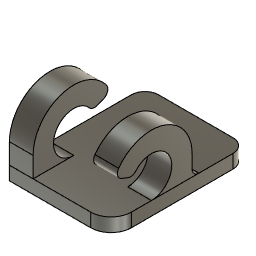
CableGuide v3 (Autodesk Fusion 360 design; units mm, degrees)
Autodesk Fusion 360 part; units mm, degrees
note: some values were not read from the file. Set by a fixed rule: which sketch regions a step uses.
sketch "Sketch1" plane through (0, 0, 0) normal (0, 0, 1) x (1, 0, 0)
  line L0 (-32.9657, 43.8587) -> (-17.9657, 43.8587)
  line L1 (-17.9657, 43.8587) -> (-17.9657, 23.8587)
  line L2 (-17.9657, 23.8587) -> (-32.9657, 23.8587)
  line L3 (-32.9657, 23.8587) -> (-32.9657, 43.8587)
  circle A0 centre (-25.4657, 38.8587) radius 2
  dimension "d1" = 15
  dimension "d2" = 20
  dimension "d3" = 4
  dimension "d4" = 7.5
  dimension "d5" = 5
  constraint horizontal L0
  constraint vertical L1
  constraint horizontal L2
  constraint vertical L3
  measures "d1" distance of L0.start L0.end
  measures "d2" distance of L0.start L2.end
  measures "d3" diameter of A0
  measures "d4" distance of L1 A0.centre
  measures "d5" distance of L0 A0.centre
extrude "Extrude1" add sketch "Sketch1" along normal blind 2 makes body 1
sketch "Sketch3" plane through (0, 0, 0) normal (1, 0, 0) x (0, 1, 0)
  circle A0 centre (27.5, 5) radius 3
  circle A1 centre (27.5, 5) radius 6
  line L0 (24.8198, 6.3478) -> (22.0216, 7.4469)
  line L1 (33.5, 5) -> (33.5, 2)
  line L2 (33.5, 2) -> (27.5, 2)
  constraint concentric A0 A1
  constraint coincident A0 L0.start
  constraint coincident A1 L0.end
  constraint coincident A1 L1.start
  constraint tangent A1 L1
  constraint vertical L1
  constraint coincident A0 L2.end
  constraint tangent A0 L2
  constraint perpendicular L1 L2
extrude "Extrude3" add sketch "Sketch3" along normal blind 3.5 separate body contours A0 A1 L0 L2 | A1 L1 L2 picked at (25.7298, 9.6652) makes body 2
move_body "Move6" bodies 2 to x (1, 0, 0) y (0, 1, 0) z (0, 0, 1) at (-22, 2, 0)
move_body "Move7" bodies 2 to x (1, 0, 0) y (0, 1, 0) z (0, 0, 1) at (0.5, 0, 0)
copy_body "CopyPasteBodies2" bodies 2 makes body 3
move_body "Move8" bodies 3 to x (-1, 0, 0) y (0, -1, 0) z (0, 0, 1) at (-52, 48.0432, 0)
move_body "Move9" bodies 3 to x (1, 0, 0) y (0, 1, 0) z (0, 0, 1) at (0, 11, 0)
move_body "Move10" bodies 3 to x (1, 0, 0) y (0, 1, 0) z (0, 0, 1) at (1, 0, 0)
move_body "Move11" bodies 3 to x (1, 0, 0) y (0, 1, 0) z (0, 0, 1) at (0.034, 0, 0)
move_body "Move12" bodies 2 to x (1, 0, 0) y (0, 1, 0) z (0, 0, 1) at (0.034, 0, 0)
move_body "Move13" bodies 2 3 to x (1, 0, 0) y (0, 1, 0) z (0, 0, 1) at (0, 0.316, 0)
combine "Combine2" operation add target body 3 tool bodies 2 1
fillet "Fillet6" radius 3 1 edges at (-17.9657, 23.8587, 1) on bodies 3
fillet "Fillet7" radius 2 2 edges at (-17.9657, 43.8587, 1) (-32.9657, 43.8587, 1) on bodies 3
fillet "Fillet8" radius 1 2 edges at (-19.716, 27.1358, 6.3478) (-19.716, 24.3376, 7.4469) on bodies 3
fillet "Fillet9" radius 1 2 edges at (-31.216, 32.5394, 6.3478) (-31.216, 35.3376, 7.4469) on bodies 3
fillet "Fillet10" radius 1 1 edges at (-19.716, 35.816, 2) on bodies 3
